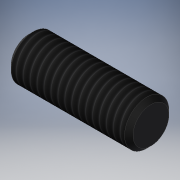
# Autodesk Inventor part: MDK 0802-302200 Shaft
Saved by Autodesk Inventor 2019 (Build 230136000, 136)
## iProperties
Created: 2024-04-08
Part Number: MDK 0802-302200 Shaft
Material: Generic
Catalog Web Link: www.cadenas.de
Description: Miniature non-preloaded type MDK-shaft-
Vendor: THK
Document SubType Name: Modeling
Designer: psAdmin
Manufacturer: THK
Mass: 1.092 g
Surface Area: 6.29336 cm^2
Volume: 1.092 cm^3
Density: 1 g/cm^3
Appearance: PSOLRGB-175-175-175
Category: PARTsolutions
Company: THK
Title: MDK 0802-302200 Shaft
Author: Cadenas PARTsolutions
PSOL_IDENT_0: {$CADENAS_DATA/23d-libs/thk/fed_screw/ball_screw/ball_screw/standard_lead_prec_gbs/miniature_mdk_1.p
PSOL_IDENT_1: rj},234 {VTYP=3D},{NB=MDK 0802-302200 Shaft},{LINA=MDK 0802-302200 Shaft},{NN=Miniature non-preloade
PSOL_IDENT_2: d type MDK-shaft},{DATE=01.04.2024 00:21:35},{GEOMDATE=26.09.2023 12:44:02},{VERSION=},{LINEID=50},{
PSOL_IDENT_3: WBVAR=ST,FS,SS,PN,SEM},{WBNUMERIC=ST,PN}  {NB=MDK 0802-302200 Shaft},{LINA=MDK 0802-302200 Shaft},{K
PSOL_IDENT_4: T=DUMMY},{IDNR=},{TP=MDK series},{MN=MDK 0802-3},{ST=0.0},{STX=268},{NOTE1=There is the groove on bo
PSOL_IDENT_5: th ends of the stroke},{FS=},{FSX='','None','H1','Type_H1','H3','Type_H3'},{SS=},{OL=22},{NOTE2=Over
PSOL_IDENT_6: all thread length is added to the both ends},{PN=0},{PNX=0},{SS1='','None','K','Type_K'},{OLX=22},{O
PSOL_IDENT_7: L3=0},{OL4=0},{D=8},{EL=290.000},{L=22.000},{E3=9.000},{A3=6.000},{F3=6.800},{B3=5.700},{G3=0.800},{
PSOL_IDENT_8: E=25.000},{F=6.000},{E1=0.000},{F1=0.000},{N=4.000},{H=4.000},{ELX=22},{FSXX=},{SS2=},{PITCH=1.250},
PSOL_IDENT_9: {LN=10.000},{A2=5.000},{B=4.000},{S2=7.000},{J=5.000},{G=0.000},{T=0.000},{P=5.000},{R=3.700},{PITCH
PSOL_IDENT_10: 3=0.500},{IP=0},{S=0.000},{SEM=0},{LEAD=0.000},{LEADX=5.000},{XA=0.000}
NB: MDK 0802-302200 Shaft
NN: Miniature non-preloaded type MDK-shaft
NBSYN: $MN.$ST.$FS.$SS.$OL.$PN.$SEM. Shaft
LINA: MDK 0802-302200 Shaft
CATALOG: THK
TP: MDK series
MN: MDK 0802-3
ST: 0
NOTE1: There is the groove on both ends of the stroke
NOTE2: Overall thread length is added to the both ends
PN: 0
D: 8
EL: 290
L: 22
E3: 9
A3: 6
F3: 6.8
B3: 5.7
G3: 0.8
E: 25
F: 6
E1: 0
F1: 0
N: 4
H: 4
PITCH: 1.25
LN: 10
A2: 5
B: 4
S2: 7
J: 5
G: 0
T: 0
P: 5
R: 3.7
PITCH3: 0.5
S: 0
SEM: 0 : without marking
LEAD: 0
LEADX: 5
SUPPLIER: THK
ARTICLENO: MDK 0802-302200 Shaft
BOMINFO: MDK 0802-302200 Shaft
CREATOR: CADENAS GmbH
Autodesk Inventor part; units mm, degrees
sketch "Sketch_2" plane through (0, 0, 0) normal (0, 0, 1) x (1, 0, 0)
  line L0 (22, 0) -> (0, 0)
  line L1 (0, 0) -> (0, 3.233)
  line L2 (0, 3.233) -> (0.767, 4)
  line L3 (0.767, 4) -> (21.233, 4)
  line L4 (21.233, 4) -> (22, 3.233)
  line L5 (22, 3.233) -> (22, 0)
  line L6 (22, 0) -> (0, 0)
  constraints: 14 end point
revolve "Revolution1" add sketch "Sketch_2" angle 360 about axis through (22, 0, 0) along (1, 0, 0)
thread "Thread1" size "M8x1.25" class "6g" standard "ISO Metric profile" full length
ref_plane "mdk_1_XY" through (0, 0, 0) normal (-1, 0, 0) x (0, 0, -1)
ref_plane "mdk_1_YZ" through (0, 0, 0) normal (0, 0, -1) x (0, -1, 0)
ref_plane "mdk_1_ZX" through (0, 0, 0) normal (0, -1, 0) x (-1, 0, 0)
ref_plane "mdk_d_XY" through (0, 0, 0) normal (0, 1, 0) x (1, 0, 0)
ref_plane "mdk_d_YZ" through (0, 0, 0) normal (1, 0, 0) x (0, 0, -1)
ref_plane "mdk_d_ZX" through (0, 0, 0) normal (0, 0, -1) x (0, 1, 0)
body "Solid1"
